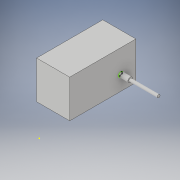
# Autodesk Inventor part: Motor_rechts
Saved by Autodesk Inventor 2019.5 (Build 235369000, 369)
## iProperties
Created: 2021-09-30
Part Number: Motor_rechts
Material: Generisch
Document SubType Name: Modeling
Designer: mritt
Density: 1 g/cm^3
Appearance: Vorgabe
Author: mritt
Autodesk Inventor part; units mm, degrees
ref_plane "YZ Plane" through (0, 0, 0) normal (1, 0, 0) x (0, 1, 0)
ref_plane "XZ Plane" through (0, 0, 0) normal (0, 1, 0) x (-1, 0, 0)
ref_plane "XY Plane" through (0, 0, 0) normal (0, 0, 1) x (1, 0, 0)
sketch "Skizze1" plane through (0, 0, 0) normal (0, 1, 0) x (-1, 0, 0)
  line L0 (48.5149, -32.0545) -> (13.5149, -32.0545)
  line L1 (13.5149, -32.0545) -> (13.5149, -102.0545)
  line L2 (13.5149, -102.0545) -> (48.5149, -102.0545)
  line L3 (48.5149, -102.0545) -> (48.5149, -32.0545)
  point P0 (0, 0)
  dimension "d0" = 70
  dimension "d1" = 35
  constraints: 8 end point, 2 parallel, 1 horizontal, 1 perpendicular
  measures "d0" distance of L0.end L1.end
  measures "d1" distance of L1.end L2.end
extrude "Extrusion1" add sketch "Skizze1" along normal blind 40
sketch "Skizze2" plane through (-13.5149, 0, -32.0545) normal (1, 0, 0) x (0, 0, -1)
  circle A0 centre (54.0519, 15.5661) radius 1.5
  circle A1 centre (54.0519, 15.5661) radius 2.5
  point P0 (-32.0545, 0)
  dimension "d4" = 3
  dimension "d5" = 5
  constraints: 2 centre point, 1 coincident
  measures "d4" diameter of A0
  measures "d5" diameter of A1
extrude "Extrusion2" add sketch "Skizze2" along normal blind 40 contours A0
extrude "Extrusion3" add sketch "Skizze2" along normal blind 10
